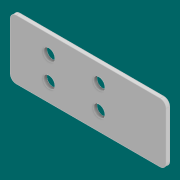
# Autodesk Inventor part: StockMountPlate
Saved by Autodesk Inventor 2020.4 (Build 244396010, 396A)
## iProperties
Created: 2022-09-13
Part Number: StockMountPlate
Material: Generic
Document SubType Name: Sheet Metal
Designer: Val
Density: 1 g/cm^3
Sheet Metal Rule: Default
Appearance: Default
Author: Val
Autodesk Inventor part; units mm, degrees
ref_plane "YZ Plane" through (0, 0, 0) normal (1, 0, 0) x (0, 1, 0)
ref_plane "XZ Plane" through (0, 0, 0) normal (0, 1, 0) x (-1, 0, 0)
ref_plane "XY Plane" through (0, 0, 0) normal (0, 0, 1) x (1, 0, 0)
sketch "Base" plane through (0, 0, 0) normal (0, 0, 1) x (1, 0, 0)
  line L0 (0, 0) -> (12.7, 0) construction
  line L1 (12.7, -15.9583) -> (-70.993, -15.9583) construction
  line L2 (12.7, 0) -> (12.7, -15.9583) construction
  line L3 (12.7, -31.9166) -> (12.7, -15.9583) construction
  line L4 (0, -31.9166) -> (12.7, -31.9166) construction
  circle A0 centre (-23.3035, -22.3083) radius 3.175
  circle A1 centre (-50.1821, -22.3083) radius 3.175
  circle A2 centre (-50.1821, -22.3083) radius 3.175
  circle A3 centre (-23.3035, -9.6083) radius 3.175
  circle A4 centre (-50.1821, -9.6083) radius 3.175
  line L5 (-50.1821, -9.6083) -> (-23.3035, -9.6083) construction
  line L6 (-50.1821, -22.3083) -> (-23.3035, -22.3083) construction
  line L7 (-50.1821, -9.6083) -> (-50.1821, -22.3083) construction
  line L8 (-23.3035, -9.6083) -> (-23.3035, -22.3083) construction
  line L9 (0, 0) -> (-70.993, 0) construction
  line L10 (0, -31.9166) -> (-70.993, -31.9166) construction
  line L11 (-70.993, -31.9166) -> (-70.993, 0) construction
  line L12 (-70.993, 0) -> (12.7, 0)
  line L13 (12.7, 0) -> (12.7, -31.9166)
  line L14 (12.7, -31.9166) -> (-70.993, -31.9166)
  line L15 (-70.993, -31.9166) -> (-70.993, 0)
  dimension "d0" = 6.35
  dimension "d1" = 6.35
  dimension "d2" = 180
  dimension "d3" = 90
  dimension "d4" = 36.0035
  dimension "d5" = 62.8821
  dimension "d6" = 83.693
  dimension "d7" = 15.9583
  dimension "d8" = 6.35
  dimension "d9" = 6.35
  dimension "d10" = 12.7
  dimension "d11" = 12.7
  dimension "d12" = 15.9583
  dimension "d13" = 0
  dimension "d14" = 12.7
  dimension "d15" = 12.7
  dimension "d16" = 62.8821
  dimension "d17" = 6.35
  measures "d0" diameter of A3
  measures "d1" diameter of A2
  measures "d2" angle of L3 L2
  measures "d3" angle of L2 L0
  measures "d4" distance between parallel lines of L3 L8
  measures "d5" distance between parallel lines of L3 L7
  measures "d6" distance between parallel lines of L3 L11
  measures "d7" distance between parallel lines of L10 L1
  measures "d8" distance between parallel lines of L1 L5
  measures "d9" distance between parallel lines of L1 L6
  measures "d10" distance from line of point (0, 0) L2
  measures "d11" distance from line of point (0, 0) L3
  measures "d12" distance from line of point (0, 0) L1
  measures "d13" distance from line of L3.end L1
  measures "d14" distance from line of L0.start L2
  measures "d15" distance from line of L4.start L2
  measures "d16" distance from line of A1.centre L2
  measures "d17" distance from line of A1.centre L1
extrude "Plate1" add sketch "Base" along normal blind 2
fillet "Corner Round1" radius 3.175 4 edges at (12.7, -31.9166, 1) (12.7, 0, 1) (-70.993, -31.9166, 1) (-70.993, 0, 1)
equation "\"d18\" = Thickness"
equation "\"BendRadius\" = Thickness"
equation "\"BendReliefWidth\" = Thickness"
equation "\"BendReliefDepth\" = 0.5 * Thickness"
equation "\"CornerReliefSize\" = 4 * Thickness"
equation "\"MinimumRemnant\" = 2 * Thickness"
equation "\"TransitionRadius\" = BendRadius"
equation "\"JacobiRadiusSize\" = BendRadius"
equation "\"GapSize\" = Thickness"
equation "\"Thickness\" = 2"
body "Solid1"
